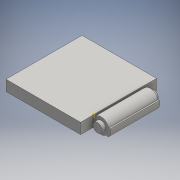
# Autodesk Inventor part: OneEdge
Saved by Autodesk Inventor 2016 (Build 200138000, 138)
## iProperties
Created: 2016-10-09
Part Number: OneEdge
Material: Generic
Document SubType Name: Modeling
Designer: Kevin
Density: 1 g/cm^3
Appearance: Default
Author: Kevin
Autodesk Inventor part; units mm, degrees
ref_plane "YZ Plane" through (0, 0, 0) normal (1, 0, 0) x (0, 1, 0)
ref_plane "XZ Plane" through (0, 0, 0) normal (0, 1, 0) x (-1, 0, 0)
ref_plane "XY Plane" through (0, 0, 0) normal (0, 0, 1) x (1, 0, 0)
sketch "Sketch1" plane through (0, 0, 0) normal (0, 0, 1) x (1, 0, 0)
  line L0 (0, 0) -> (530.86, 0)
  line L1 (530.86, 0) -> (530.86, -541.02)
  line L2 (530.86, -541.02) -> (0, -541.02)
  line L3 (0, -541.02) -> (0, 0)
  dimension "d0" = 530.86
  dimension "d1" = 541.02
  constraints: 8 end point, 2 parallel, 1 horizontal, 1 perpendicular
  measures "d0" distance of L1.end L2.end
  measures "d1" distance of L0.end L1.end
extrude "Extrusion1" add sketch "Sketch1" along normal blind 76.2
ref_plane "Work Plane1" through (530.86, -450.59, 76.2) normal (0, -1, 0) x (1, 0, 0)
sketch "Sketch5" plane through (530.86, -450.59, 76.2) normal (0, -1, 0) x (1, 0, 0)
  line L0 (0, -76.2) -> (0, 0) projected
  line L1 (0, -76.2) -> (0, -38.1)
  line L2 (0, -38.1) -> (55, -38.1)
  circle A0 centre (55, -38.1) radius 55
  arc A1 (94.666, -76.2) -> (110, -38.1) centre (55, -38.1) ccw
  arc A2 (94.666, -76.2) -> (108.9585, -27.4475) centre (55, -38.1) ccw
  line L3 (94.666, -76.2) -> (104.1299, -84.366)
  line L4 (108.9585, -27.4475) -> (121.1714, -24.7835)
  arc A3 (104.1299, -84.366) -> (121.1714, -24.7835) centre (65.3605, -41.0491) ccw
  point P0 (-530.86, -76.2)
  dimension "d13" = 38.1
  dimension "d14" = 55
  dimension "d15" = 110
  dimension "d18" = 12.5
  dimension "d19" = 12.5
  constraints: 10 point on circle, 8 end point, 4 centre point, 3 concentric, 1 coincident, 1 midpoint, 1 perpendicular
  measures "d13" distance of L0.start L1.end
  measures "d14" distance of L1.end L2.end
  measures "d15" diameter of A0
  measures "d18" distance of L3.start L3.end
  measures "d19" distance of L4.start L4.end
extrude "Extrusion4" add sketch "Sketch5" against normal blind 350
sketch "Sketch6" plane through (530.86, -450.59, 76.2) normal (0, -1, 0) x (1, 0, 0)
  arc A0 (0, -38.1) -> (94.666, -76.2) centre (55, -38.1) ccw projected
  circle A1 centre (55, -38.1) radius 32.5
  point P0 (-530.86, -76.2)
  dimension "d20" = 65
  constraints: 1 centre point, 1 coincident
  measures "d20" diameter of A1
extrude "Extrusion5" add sketch "Sketch6" along normal blind 25
sketch "Sketch7" plane through (530.86, -100.59, 76.2) normal (0, 1, 0) x (1, 0, 0)
  arc A0 (94.666, 76.2) -> (0, 38.1) centre (55, 38.1) ccw projected
  line L0 (94.666, 76.2) -> (55, 38.1)
  line L1 (0, 38.1) -> (55, 38.1)
  circle A1 centre (55, 38.1) radius 32.5
  point P0 (-530.86, 76.2)
  constraints: 4 end point, 1 centre point, 1 coincident, 1 horizontal
extrude "Extrusion6" add sketch "Sketch7" along normal blind 25 contours A1 L1 L0 | L0 L1 A1
body "Solid1"
